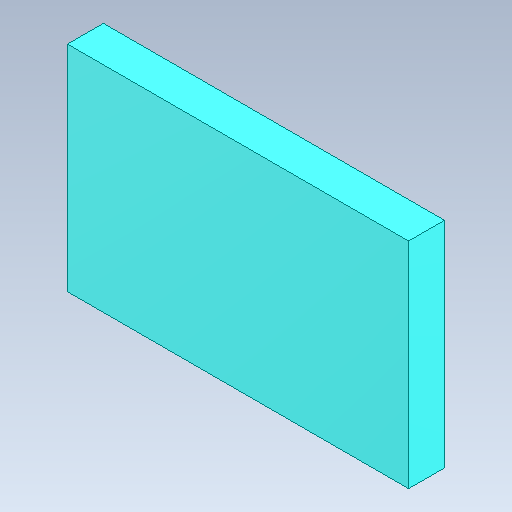
# Autodesk Inventor part: TB6612FNG
Saved by Autodesk Inventor 2020 (Build 240168000, 168)
## iProperties
Created: 2019-05-24
Part Number: TB6612FNG
Material: Generic
Document SubType Name: Modeling
Designer: psrob
Density: 1 g/cm^3
Appearance: SSOP24, TB6612FNG
Author: psrob
Autodesk Inventor part; units mm, degrees
ref_plane "YZ Plane" through (0, 0, 0) normal (1, 0, 0) x (0, 1, 0)
ref_plane "XZ Plane" through (0, 0, 0) normal (0, 1, 0) x (-1, 0, 0)
ref_plane "XY Plane" through (0, 0, 0) normal (0, 0, 1) x (1, 0, 0)
sketch "SSOP24, TB6612FNG_56" plane through (0, 0, 0) normal (0, 0, 1) x (1, 0, 0)
  line L0 (-5.1507, 2.6016) -> (4.3516, 2.6016)
  line L1 (4.3516, 2.6016) -> (4.3516, -3.3727)
  line L2 (4.3516, -3.3727) -> (-5.1507, -3.3727)
  line L3 (-5.1507, -3.3727) -> (-5.1507, 2.6016)
  constraints: 8 end point
extrude "Extrusion1" add sketch "SSOP24, TB6612FNG_56" along normal blind 1
body "Solid1"
